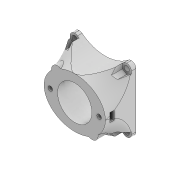
# Autodesk Inventor part: Female 22 to oxy
Saved by Autodesk Inventor 2020 (Build 240168000, 168)
## iProperties
Created: 2020-05-08
Part Number: Female 22 to oxy
Material: Generic
Document SubType Name: Modeling
Designer: rayan
Density: 1 g/cm^3
Appearance: Default
Author: rayan
Autodesk Inventor part; units mm, degrees
ref_plane "YZ Plane" through (0, 0, 0) normal (1, 0, 0) x (0, 1, 0)
ref_plane "XZ Plane" through (0, 0, 0) normal (0, 1, 0) x (-1, 0, 0)
ref_plane "XY Plane" through (0, 0, 0) normal (0, 0, 1) x (1, 0, 0)
sketch "Sketch3" plane through (0, 0, 0) normal (0, 0, 1) x (1, 0, 0)
  line L0 (-20.1, 21) -> (20.1, 21)
  line L1 (20.1, 21) -> (20.1, -21)
  line L2 (20.1, -21) -> (-20.1, -21)
  line L3 (-20.1, -21) -> (-20.1, 21)
  line L4 (-20.1, 21) -> (20.1, -21) construction
  line L5 (20.1, 21) -> (-20.1, -21) construction
  point P0 (0, 0)
  dimension "d24" = 40.2
  dimension "d25" = 42
  constraints: 12 end point, 2 midpoint, 2 parallel, 1 horizontal, 1 perpendicular
  measures "d24" distance of L1.end L2.end
  measures "d25" distance of L0.end L1.end
extrude "Extrusion3" add sketch "Sketch3" along normal blind 20
sketch "Sketch4" plane through (0, 0, 20) normal (0, 0, 1) x (1, 0, 0)
  line L0 (20.1, 21) -> (-20.1, 21) projected
  line L1 (-20.1, 21) -> (-17.1, 21) construction
  line L2 (-17.1, 21) -> (-17.1, 18) construction
  line L3 (-17.1, 18) -> (-20.1, 18) construction
  line L4 (-20.1, 18) -> (-20.1, 21) construction
  circle A0 centre (-17.1, 18) radius 1.7
  point P0 (0, 0)
  dimension "d28" = 3
  dimension "d29" = 3
  dimension "d30" = 3.4
  constraints: 8 end point, 2 parallel, 1 centre point, 1 coincident, 1 horizontal, 1 perpendicular
  measures "d28" distance of L2.end L3.end
  measures "d29" distance of L1.end L2.end
  measures "d30" diameter of A0
extrude "Extrusion4" cut sketch "Sketch4" against normal through all
fillet "Fillet2" radius 3 1 edges at (-20.1, 21, 10)
mirror "Mirror2" about plane through (0, 0, 0) normal (0, 1, 0) of "Fillet2", "Extrusion4"
mirror "Mirror3" about plane through (0, 0, 0) normal (1, 0, 0) of "Fillet2", "Extrusion4", "Mirror2"
sketch "Sketch5" plane through (0, 0, 20) normal (0, 0, 1) x (1, 0, 0)
  circle A0 centre (-17.1, 18) radius 1.7 construction
  circle A1 centre (17.1, 18) radius 1.7 construction
  line L0 (-17.1, 18) -> (17.1, 18) construction
  line L1 (17.1, 18) -> (17.1, 15) construction
  line L2 (17.1, 15) -> (-17.1, 15) construction
  line L3 (-17.1, 15) -> (-17.1, 18) construction
  arc A2 (-17.1, 21) -> (-20.1, 18) centre (-17.1, 18) ccw construction
  line L4 (-17.1, 18) -> (-17.1, 21) construction
  line L5 (17.1, 21) -> (-17.1, 21) construction
  line L6 (17.1, 18) -> (17.1, 21) construction
  line L7 (-17.1, 18) -> (-17.1, 21) construction
  line L8 (-17.1, 21) -> (-16, 21) construction
  line L9 (-16, 21) -> (-16, 18) construction
  line L10 (-16, 18) -> (-17.1, 18) construction
  line L11 (17.1, 18) -> (17.1, 21) construction
  line L12 (17.1, 21) -> (16, 21) construction
  line L13 (16, 21) -> (16, 18) construction
  line L14 (16, 18) -> (17.1, 18) construction
  arc A3 (-16, 21) -> (16, 21) centre (0, 39.3333) ccw
  line L15 (-16, 21) -> (16, 21)
  point P0 (0, 0)
  point P1 (0, 15)
  dimension "d34" = 3
  dimension "d87" = 1.1
  dimension "d88" = 1.1
  constraints: 30 end point, 7 equal length, 5 perpendicular, 3 point on circle, 2 vertical, 1 centre point, 1 horizontal, 1 midpoint
  measures "d34" distance of L0.end L1.end
  measures "d87" distance of L4.end L8.end
  measures "d88" distance of L13.end L0.end
extrude "Extrusion5" cut sketch "Sketch5" against normal through all
mirror "Mirror4" about plane through (0, 0, 0) normal (0, 1, 0) of "Extrusion5"
fillet "Fillet3" radius 3 4 edges at (16, 21, 10) (-16, 21, 10) (-16, -21, 10) (16, -21, 10)
sketch "Sketch7" plane through (0, 0, 20) normal (0, 0, 1) x (1, 0, 0)
  line L0 (15.3, 7.9) -> (15.3, -11.6) construction
  line L1 (15.3, -11.6) -> (-15.4, -11.6) construction
  line L2 (-15.4, -11.6) -> (-15.4, 7.9) construction
  line L3 (-15.4, 7.9) -> (15.3, 7.9) construction
  line L4 (-17.65, -15) -> (30.6, -15) construction
  line L5 (30.6, -15) -> (30.6, 15) construction
  line L6 (30.6, 15) -> (-30.1, 15) construction
  line L7 (-30.1, 15) -> (-30.1, 10) construction
  line L8 (-17.65, 10) -> (-30.1, 10) construction
  line L9 (-17.65, 10) -> (-17.65, -15) construction
  line L10 (15.3, -11.6) -> (-15.4, 7.9) construction
  line L11 (-15.4, -11.6) -> (15.3, 7.9) construction
  line L12 (0, 0) -> (-0.05, 0) construction
  line L13 (-0.05, 0) -> (-0.05, -1.85) construction
  line L14 (-0.05, -1.85) -> (0, -1.85) construction
  line L15 (0, -1.85) -> (0, 0) construction
  circle A0 centre (0, -1.85) radius 9
  dimension "d41" = 18
  constraints: 12 end point, 2 parallel, 1 centre point, 1 coincident, 1 horizontal, 1 midpoint, 1 perpendicular
  measures "d41" diameter of A0
extrude "Extrusion6" cut sketch "Sketch7" against normal through all
sketch "Sketch8" plane through (0, 0, 0) normal (1, 0, 0) x (0, 1, 0)
  line L0 (7.15, 0) -> (-10.85, 0) projected
  line L1 (-10.85, 20) -> (7.15, 20) projected
  line L2 (-18, 0) -> (18, 0) projected
  line L3 (-18, 20) -> (18, 20) projected
  line L4 (-1.45, 0) -> (-1.45, 20)
  line L5 (-1.45, 20) -> (9.55, 20)
  line L6 (9.55, 20) -> (9.55, 0) construction
  line L7 (9.55, 0) -> (-1.45, 0)
  line L8 (0, 0) -> (-1.45, 0)
  line L9 (9.55, 0) -> (9.55, 20) construction
  line L10 (9.55, 20) -> (9.8, 20) construction
  line L11 (9.8, 20) -> (9.8, 0) construction
  line L12 (9.8, 0) -> (9.55, 0) construction
  line L13 (9.55, 0) -> (9.8, 20)
  line L14 (9.55, 20) -> (9.8, 20)
  point P0 (-17.2722, 0)
  point P1 (17.2722, 0)
  point P2 (-17.2722, 20)
  point P3 (17.2722, 20)
  point P4 (9.8, 20)
  dimension "d42" = 11
  dimension "d43" = 0.25
  constraints: 22 end point, 4 parallel, 3 collinear, 3 perpendicular, 2 point on line
  measures "d42" distance of L4.end L5.end
  measures "d43" distance of L5.end L10.end
revolve "Revolution1" cut sketch "Sketch8" angle 360 about axis through (0, -1.45, 0) along (0, 0, 1)
sketch "Sketch9" plane through (0, 0, 20) normal (0, 0, 1) x (1, 0, 0)
  line L0 (6.3337, 11.8636) -> (-10.8812, 11.8636) construction
  line L1 (-10.8812, 11.8636) -> (-10.8812, 17.151) construction
  line L2 (-10.8812, 17.151) -> (6.3337, 17.151) construction
  line L3 (6.3337, 17.151) -> (6.3337, 11.8636) construction
  point P0 (0, 0)
  constraints: 2 other
extrude "Extrusion7" [suppressed]
ref_plane "Work Plane1" through (0, 0, 3) normal (0, 0, -1) x (-1, 0, 0)
sketch "Sketch10" plane through (0, 0, 3) normal (0, 0, -1) x (-1, 0, 0)
  circle A0 centre (-17.1, -18) radius 1.7 construction
  line L0 (-17.1, -18) -> (-17.1, -23.7125) construction
  line L1 (-17.1, -21.3486) -> (-20, -19.6743) construction
  line L2 (-20, -19.6743) -> (-20, -16.3257) construction
  line L3 (-20.1, -16.3834) -> (-17.1, -14.6514)
  line L4 (-17.1, -14.6514) -> (-14.2, -16.3257)
  line L5 (-14.2, -16.3257) -> (-14.2, -19.6743)
  line L6 (-14.2, -19.6743) -> (-17.1, -21.3486) construction
  line L7 (-14.2, -19.6743) -> (-20, -19.6743) construction
  line L8 (-20, -19.6743) -> (-20, -21.4064) construction
  line L9 (-20, -21.4064) -> (-14.2, -21.4064)
  line L10 (-14.2, -21.4064) -> (-14.2, -19.6743)
  circle A1 centre (0, -1.45) radius 11 construction
  arc A2 (-17.088, -21) -> (-15.2125, -20.3415) centre (-17.088, -18) ccw construction
  arc A3 (15.2125, -20.3415) -> (-15.2125, -20.3415) centre (0, -39.3333) ccw construction
  arc A4 (15.2125, -20.3415) -> (17.088, -21) centre (17.088, -18) ccw construction
  line L11 (17.1, -21) -> (17.088, -21) construction
  arc A5 (17.1, -21) -> (20.1, -18) centre (17.1, -18) ccw construction
  line L12 (20.1, 18) -> (20.1, -18) construction
  arc A6 (20.1, 18) -> (17.1, 21) centre (17.1, 18) ccw construction
  line L13 (17.088, 21) -> (17.1, 21) construction
  arc A7 (17.088, 21) -> (15.2125, 20.3415) centre (17.088, 18) ccw construction
  arc A8 (-15.2125, 20.3415) -> (15.2125, 20.3415) centre (0, 39.3333) ccw construction
  arc A9 (-15.2125, 20.3415) -> (-17.088, 21) centre (-17.088, 18) ccw construction
  line L14 (-17.1, 21) -> (-17.088, 21) construction
  arc A10 (-17.1, 21) -> (-20.1, 18) centre (-17.1, 18) ccw construction
  line L15 (-20.1, -18) -> (-20.1, 18) construction
  arc A11 (-20.1, -18) -> (-17.1, -21) centre (-17.1, -18) ccw construction
  line L16 (-17.088, -21) -> (-17.1, -21) construction
  circle A12 centre (-17.1, 18) radius 1.7 construction
  circle A13 centre (17.1, 18) radius 1.7 construction
  circle A14 centre (17.1, -18) radius 1.7 construction
  circle A15 centre (-17.1, -18) radius 1.7 construction
  line L17 (-20.1, -16.3834) -> (-20, -16.3834) construction
  line L18 (-20, -16.3834) -> (-20, -21.4064) construction
  line L19 (-20, -21.4064) -> (-20.1, -21.4064)
  line L20 (-20.1, -21.4064) -> (-20.1, -16.3834)
  point P0 (0, 0)
  dimension "d48" = 5.8
  constraints: 30 end point, 4 parallel, 3 point on line, 2 horizontal, 2 perpendicular, 1 coincident, 1 vertical, 13 other
  measures "d48" distance between parallel lines of L2 L5
extrude "Extrusion8" cut sketch "Sketch10" against normal through all
mirror "Mirror5" about plane through (0, 0, 0) normal (0, 1, 0) of "Extrusion8"
mirror "Mirror6" about plane through (0, 0, 0) normal (1, 0, 0) of "Extrusion8", "Mirror5"
sketch "Sketch11" plane through (0, 0, 20) normal (0, 0, 1) x (1, 0, 0)
  circle A0 centre (0, -1.45) radius 11.25 projected
  line L0 (0, -1.45) -> (16, -1.45)
  line L1 (20.1, -18) -> (20.1, 18) projected
  circle A1 centre (16, -1.45) radius 1.5
  point P0 (0, 0)
  point P1 (20.1, -17.2722)
  point P2 (20.1, 17.2722)
  dimension "d51" = 16
  dimension "d52" = 3
  constraints: 2 end point, 1 centre point, 1 coincident, 1 perpendicular
  measures "d51" distance of L0.start L0.end
  measures "d52" diameter of A1
extrude "Extrusion9" cut sketch "Sketch11" against normal blind 10 contours A1
ref_plane "Work Plane2" through (0, 0, 17) normal (0, 0, 1) x (1, 0, 0)
sketch "Sketch12" plane through (0, 0, 17) normal (0, 0, 1) x (1, 0, 0)
  circle A0 centre (16, -1.45) radius 1.5 projected
  line L0 (16, -1.45) -> (21, -1.45)
  line L1 (19.3486, -1.45) -> (17.6743, -4.35) construction
  line L2 (17.6743, -4.35) -> (14.3257, -4.35)
  line L3 (14.3257, -4.35) -> (12.6514, -1.45)
  line L4 (12.6514, -1.45) -> (14.3257, 1.45)
  line L5 (14.3257, 1.45) -> (17.6743, 1.45)
  line L6 (17.6743, 1.45) -> (19.3486, -1.45) construction
  line L7 (17.6743, -4.35) -> (17.6743, 1.45) construction
  line L8 (17.6743, 1.45) -> (27.6743, 1.45)
  line L9 (27.6743, 1.45) -> (27.6743, -4.35)
  line L10 (27.6743, -4.35) -> (17.6743, -4.35)
  point P0 (0, 0)
  point P1 (16, -1.85)
  dimension "d111" = 5
  dimension "d112" = 5.8
  dimension "d113" = 10
  constraints: 22 end point, 2 parallel, 2 perpendicular, 1 coincident, 1 horizontal, 1 point on line, 13 other
  measures "d111" distance of L0.start L0.end
  measures "d112" distance between parallel lines of L2 L5
  measures "d113" distance of L9.end L1.end
extrude "Extrusion10" cut sketch "Sketch12" against normal blind 2.8
mirror "Mirror7" about plane through (0, 0, 0) normal (1, 0, 0) of "Extrusion10", "Extrusion9"
sketch "Sketch13" plane through (0, 0, 20) normal (0, 0, 1) x (1, 0, 0)
  circle A0 centre (-17.1, 18) radius 1.7 projected
  point P0 (0, 0)
extrude "Extrusion11" [suppressed]
mirror "Mirror8" [suppressed]
mirror "Mirror9" [suppressed]
sketch "Sketch14" plane through (0, 0, 0) normal (0, 0, -1) x (-1, 0, 0)
  line L0 (5.3455, 10.4926) -> (-17.7314, 10.4926) construction
  line L1 (-17.7314, 10.4926) -> (-17.7314, 22.1476) construction
  line L2 (-17.7314, 22.1476) -> (5.3455, 22.1476) construction
  line L3 (5.3455, 22.1476) -> (5.3455, 10.4926) construction
  spline S0 degree 2 poles (2.9398, 12.6949) (2.9398, 12.8381) (3.0114, 13.0787) (3.1432, 13.2734) (3.3293, 13.4166) (3.5613, 13.5169) (3.8276, 13.5656) (3.9995, 13.5656) knots 0 0 0 1 2 3 4 5 6 6 6
  line L4 (3.9995, 13.5656) -> (4.7927, 13.5656)
  spline S1 degree 2 poles (4.7927, 13.5656) (4.8443, 13.5656) (4.9417, 13.494) (4.9417, 13.4023) knots 0 0 0 1 2 2 2
  line L5 (4.9417, 13.4023) -> (4.9417, 10.6931)
  spline S2 degree 2 poles (4.9417, 10.6931) (4.9417, 10.6015) (4.8443, 10.5299) (4.7927, 10.5299) knots 0 0 0 1 2 2 2
  line L6 (4.7927, 10.5299) -> (4.1025, 10.5299)
  spline S3 degree 2 poles (4.1025, 10.5299) (3.8276, 10.5299) (3.4811, 10.633) (3.2491, 10.8306) (3.1317, 11.117) (3.1317, 11.2974) knots 0 0 0 1 2 3 4 4 4
  spline S4 degree 2 poles (3.1317, 11.2974) (3.1317, 11.4062) (3.1833, 11.601) (3.2835, 11.7699) (3.4381, 11.8988) (3.5355, 11.9417) knots 0 0 0 1 2 3 4 4 4
  spline S5 degree 2 poles (3.5355, 11.9417) (3.4124, 11.9647) (3.1947, 12.0907) (3.0343, 12.2825) (2.9398, 12.5403) (2.9398, 12.6949) knots 0 0 0 1 2 3 4 4 4
  spline S6 degree 2 poles (3.3637, 12.7179) (3.3637, 12.5833) (3.4496, 12.3771) (3.6157, 12.2339) (3.8677, 12.1623) (4.0567, 12.1623) knots 0 0 0 1 2 3 4 4 4
  line L7 (4.0567, 12.1623) -> (4.5407, 12.1623)
  line L8 (4.5407, 12.1623) -> (4.5407, 13.2333)
  line L9 (4.5407, 13.2333) -> (3.9536, 13.2333)
  spline S7 degree 2 poles (3.9536, 13.2333) (3.8162, 13.2333) (3.61, 13.1675) (3.4525, 13.0386) (3.3637, 12.8467) (3.3637, 12.7179) knots 0 0 0 1 2 3 4 4 4
  spline S8 degree 2 poles (3.547, 11.3375) (3.547, 11.2286) (3.6071, 11.0482) (3.7388, 10.9251) (3.9508, 10.8592) (4.1226, 10.8592) knots 0 0 0 1 2 3 4 4 4
  line L10 (4.1226, 10.8592) -> (4.5407, 10.8592)
  line L11 (4.5407, 10.8592) -> (4.5407, 11.8415)
  line L12 (4.5407, 11.8415) -> (4.0825, 11.8415)
  spline S9 degree 2 poles (4.0825, 11.8415) (3.925, 11.8415) (3.7331, 11.7585) (3.6042, 11.621) (3.547, 11.4348) (3.547, 11.3375) knots 0 0 0 1 2 3 4 4 4
  spline S10 degree 2 poles (0.0531, 13.4224) (0.0359, 13.4739) (0.033, 13.5369) (0.0702, 13.5713) (0.1562, 13.5799) (0.2306, 13.5799) knots 0 0 0 1 2 3 4 4 4
  spline S11 degree 2 poles (0.2306, 13.5799) (0.3022, 13.5799) (0.3881, 13.5741) (0.434, 13.557) (0.454, 13.5283) (0.4655, 13.5083) knots 0 0 0 1 2 3 4 4 4
  line L13 (0.4655, 13.5083) -> (0.7232, 12.7694)
  line L14 (0.7232, 12.7694) -> (1.9862, 12.7694)
  line L15 (1.9862, 12.7694) -> (2.2353, 13.4968)
  spline S12 degree 2 poles (2.2353, 13.4968) (2.2439, 13.5197) (2.2668, 13.5484) (2.3098, 13.5713) (2.3928, 13.5799) (2.4587, 13.5799) knots 0 0 0 1 2 3 4 4 4
  spline S13 degree 2 poles (2.4587, 13.5799) (2.5274, 13.5799) (2.6133, 13.5684) (2.6477, 13.534) (2.6448, 13.471) (2.6277, 13.4195) knots 0 0 0 1 2 3 4 4 4
  line L16 (2.6277, 13.4195) -> (1.6081, 10.6015)
  spline S14 degree 2 poles (1.6081, 10.6015) (1.5995, 10.5728) (1.568, 10.5413) (1.5108, 10.5213) (1.4191, 10.5156) (1.3475, 10.5156) knots 0 0 0 1 2 3 4 4 4
  spline S15 degree 2 poles (1.3475, 10.5156) (1.2731, 10.5156) (1.1757, 10.5213) (1.1127, 10.5413) (1.0812, 10.5757) (1.0726, 10.6015) knots 0 0 0 1 2 3 4 4 4
  line L17 (1.0726, 10.6015) -> (0.0531, 13.4224)
  line L18 (1.359, 10.9337) -> (1.3618, 10.9337)
  line L19 (1.3618, 10.9337) -> (1.8859, 12.4486)
  line L20 (1.8859, 12.4486) -> (0.8292, 12.4486)
  line L21 (0.8292, 12.4486) -> (1.359, 10.9337)
  spline S16 degree 2 poles (-2.4814, 13.1331) (-2.4814, 13.1703) (-2.4757, 13.2276) (-2.4643, 13.2706) (-2.4471, 13.3021) (-2.3984, 13.3508) (-2.2495, 13.4453) (-2.0261, 13.5398) (-1.7368, 13.6028) (-1.565, 13.6028) knots 0 0 0 1 2 3 4 5 6 7 8 8 8
  spline S17 degree 2 poles (-1.565, 13.6028) (-1.27, 13.6028) (-0.7918, 13.4052) (-0.4567, 13.0214) (-0.2763, 12.4544) (-0.2763, 12.0878) knots 0 0 0 1 2 3 4 4 4
  spline S18 degree 2 poles (-0.2763, 12.0878) (-0.2763, 11.7098) (-0.471, 11.1198) (-0.8233, 10.7074) (-1.3159, 10.4926) (-1.6137, 10.4926) knots 0 0 0 1 2 3 4 4 4
  spline S19 degree 2 poles (-1.6137, 10.4926) (-1.7454, 10.4926) (-1.9946, 10.5413) (-2.2036, 10.6158) (-2.3698, 10.716) (-2.4328, 10.779) (-2.4499, 10.8105) (-2.4643, 10.8563) (-2.47, 10.9165) (-2.47, 10.9594) knots 0 0 0 1 2 3 4 5 6 7 8 8 8
  spline S20 degree 2 poles (-2.47, 10.9594) (-2.47, 11.0053) (-2.4614, 11.0711) (-2.4413, 11.117) (-2.4156, 11.137) (-2.3955, 11.137) knots 0 0 0 1 2 3 4 4 4
  spline S21 degree 2 poles (-2.3955, 11.137) (-2.364, 11.137) (-2.2466, 11.0454) (-2.0576, 10.9365) (-1.7913, 10.8449) (-1.6051, 10.8449) knots 0 0 0 1 2 3 4 4 4
  spline S22 degree 2 poles (-1.6051, 10.8449) (-1.4018, 10.8449) (-1.0696, 11.0053) (-0.8319, 11.3203) (-0.703, 11.7728) (-0.703, 12.0649) knots 0 0 0 1 2 3 4 4 4
  spline S23 degree 2 poles (-0.703, 12.0649) (-0.703, 12.3513) (-0.829, 12.7952) (-1.061, 13.093) (-1.4018, 13.2448) (-1.6166, 13.2448) knots 0 0 0 1 2 3 4 4 4
  spline S24 degree 2 poles (-1.6166, 13.2448) (-1.7998, 13.2448) (-2.0719, 13.156) (-2.2609, 13.0443) (-2.3841, 12.9556) (-2.4213, 12.9556) knots 0 0 0 1 2 3 4 4 4
  spline S25 degree 2 poles (-2.4213, 12.9556) (-2.4356, 12.9556) (-2.4614, 12.9699) (-2.4757, 13.01) (-2.4814, 13.0787) (-2.4814, 13.1331) knots 0 0 0 1 2 3 4 4 4
  spline S26 degree 2 poles (-4.9988, 13.4997) (-4.9988, 13.5197) (-4.9816, 13.5484) (-4.9329, 13.5684) (-4.8556, 13.5799) (-4.7897, 13.5799) knots 0 0 0 1 2 3 4 4 4
  spline S27 degree 2 poles (-4.7897, 13.5799) (-4.7095, 13.5799) (-4.6064, 13.5656) (-4.5549, 13.5283) (-4.5377, 13.5054) knots 0 0 0 1 2 3 3 3
  line L22 (-4.5377, 13.5054) -> (-3.4208, 11.9876)
  line L23 (-3.4208, 11.9876) -> (-3.4208, 13.5054)
  spline S28 degree 2 poles (-3.4208, 13.5054) (-3.4208, 13.5226) (-3.4007, 13.5512) (-3.3549, 13.5684) (-3.2776, 13.5799) (-3.2203, 13.5799) knots 0 0 0 1 2 3 4 4 4
  spline S29 degree 2 poles (-3.2203, 13.5799) (-3.163, 13.5799) (-3.0829, 13.5684) (-3.037, 13.5512) (-3.017, 13.5226) (-3.017, 13.5054) knots 0 0 0 1 2 3 4 4 4
  line L24 (-3.017, 13.5054) -> (-3.017, 10.59)
  spline S30 degree 2 poles (-3.017, 10.59) (-3.017, 10.5728) (-3.037, 10.5442) (-3.0829, 10.527) (-3.163, 10.5156) (-3.2203, 10.5156) knots 0 0 0 1 2 3 4 4 4
  spline S31 degree 2 poles (-3.2203, 10.5156) (-3.2776, 10.5156) (-3.3549, 10.527) (-3.4007, 10.5442) (-3.4208, 10.5728) (-3.4208, 10.59) knots 0 0 0 1 2 3 4 4 4
  line L25 (-3.4208, 10.59) -> (-3.4208, 11.9389)
  line L26 (-3.4208, 11.9389) -> (-4.4947, 10.59)
  spline S32 degree 2 poles (-4.4947, 10.59) (-4.509, 10.57) (-4.5463, 10.5413) (-4.6007, 10.5241) (-4.678, 10.5156) (-4.7382, 10.5156) knots 0 0 0 1 2 3 4 4 4
  spline S33 degree 2 poles (-4.7382, 10.5156) (-4.8012, 10.5156) (-4.8756, 10.527) (-4.9214, 10.5471) (-4.9358, 10.5728) (-4.9358, 10.59) knots 0 0 0 1 2 3 4 4 4
  spline S34 degree 2 poles (-4.9358, 10.59) (-4.9358, 10.6215) (-4.9071, 10.6817) (-4.8642, 10.7361) knots 0 0 0 1 2 2 2
  line L27 (-4.8642, 10.7361) -> (-3.8561, 11.9389)
  line L28 (-3.8561, 11.9389) -> (-4.9415, 13.3794)
  spline S35 degree 2 poles (-4.9415, 13.3794) (-4.9816, 13.4424) (-4.9988, 13.4854) (-4.9988, 13.4997) knots 0 0 0 1 2 2 2
  point P0 (0, 0)
  constraints: 2 other
extrude "Extrusion12" cut sketch "Sketch14" against normal blind 0.5
sketch "Sketch26" plane through (0, 0, 20) normal (0, 0, 1) x (1, 0, 0)
  circle A0 centre (-16, -1.45) radius 1.5 projected
  circle A1 centre (16, -1.45) radius 1.5 projected
  line L0 (-20.1, 16.3834) -> (-20.1, -16.3834) projected
  arc A2 (14.2, -19.573) -> (-14.2, -19.573) centre (0, -39.3333) ccw projected
  line L1 (20.1, -16.3834) -> (20.1, 16.3834) projected
  arc A3 (-14.2, 19.573) -> (14.2, 19.573) centre (0, 39.3333) ccw projected
  circle A4 centre (0, -1.45) radius 11.25 construction
  line L2 (-16, -1.45) -> (-20.1, -1.45)
  ellipse E0 centre (0, -1.45) end of major axis (-20.1, -1.45) minor radius 16.45
  line L3 (-20.1, 16.3834) -> (-20.1, -16.3834) projected
  arc A5 (-14.2, 19.573) -> (14.2, 19.573) centre (0, 39.3333) ccw projected
  arc A6 (14.2, -19.573) -> (-14.2, -19.573) centre (0, -39.3333) ccw projected
  line L4 (0, -15) -> (0, -17.9) construction
  line L5 (-17.1, 14.6514) -> (-20.1, 16.3834) projected
  line L6 (-20.1, -16.3834) -> (-17.1, -14.6514) projected
  line L7 (-17.1, -14.6514) -> (-14.2, -16.3257) projected
  line L8 (-14.2, -16.3257) -> (-14.2, -19.573) projected
  line L9 (14.2, -19.573) -> (14.2, -16.3257) projected
  line L10 (14.2, -16.3257) -> (17.1, -14.6514) projected
  line L11 (17.1, -14.6514) -> (20.1, -16.3834) projected
  line L12 (20.1, 16.3834) -> (17.1, 14.6514) projected
  line L13 (17.1, 14.6514) -> (14.2, 16.3257) projected
  line L14 (14.2, 16.3257) -> (14.2, 19.573) projected
  line L15 (-14.2, 19.573) -> (-14.2, 16.3257) projected
  line L16 (-14.2, 16.3257) -> (-17.1, 14.6514) projected
  point P0 (0, 0)
  point P1 (0, 15)
  point P2 (0, 15)
  point P3 (20.1, -1.45)
  point P4 (-8.2627, -16.4458)
  point P5 (8.2627, -16.4458)
  constraints: 4 end point, 4 point on circle, 2 vertical, 1 coincident, 1 perpendicular, 1 point on line, 5 other
sketch "Sketch27" plane through (20.1, -18, 0) normal (1, 0, 0) x (0, 0, -1)
  line L0 (-20, 15.05) -> (-20, 18.05) projected
  line L1 (-20, 39) -> (0, 39) projected
  arc A0 (-20, 16.55) -> (-3, 39) centre (-27.9689, 40.2459) ccw
  point P0 (0, 18)
  dimension "d92" = 25
  constraints: 2 point on circle, 1 centre point, 1 midpoint
  measures "d92" radius of A0
sweep "Sweep4" cut profiles "Sketch26" path "Sketch27" keep normal constant yes path curves A0 contours L5 L16 L15 A3 E0 L0 | A3 L14 L13 L12 L1 E0
sketch "Sketch29" plane through (0, 0, 0) normal (1, 0, 0) x (0, 1, 0)
  line L0 (-15, 0) -> (-15, 20) construction
  line L1 (15, 20) -> (-17.9, 20) construction
  line L2 (-15, 20) -> (-17.9, 20) construction
  line L3 (-15, 0) -> (-20.3415, 0) construction
  line L4 (-15, 0) -> (-17.9, 20)
  point P0 (0, 0)
  constraints: 2 end point
sweep "Sweep5" add profiles "Sketch26" path "Sketch29" keep normal constant yes picked at (0.9346, -16.8782) contours A2 E0
sketch "Sketch30" plane through (-20.1, -18, 0) normal (-1, 0, 0) x (0, 0, 1)
  line L0 (20, 16.55) -> (20, 1.6166) construction
  line L1 (3, 0) -> (3, -3) projected
  arc A0 (20, 16.55) -> (3, -3) centre (22.9987, -3.2239) ccw
  point P0 (0, 18)
  dimension "d98" = 20
  constraints: 2 point on circle, 1 centre point
  measures "d98" radius of A0
sketch "Sketch31" plane through (0, 0, 20) normal (0, 0, 1) x (1, 0, 0)
  ellipse E0 centre (0, -1.45) end of major axis (20.1, -1.45) minor radius 16.45 (0, 15) -> (-20.1, -1.45) ccw projected
  line L0 (-20.1, -1.45) -> (-20.1, -16.3834) projected
  line L1 (-20.1, -16.3834) -> (-17.1, -14.6514) projected
  line L2 (-17.1, -14.6514) -> (-14.2, -16.3257) projected
  line L3 (-14.2, -16.3257) -> (-14.2, -19.573) projected
  arc A0 (-8.2627, -16.4458) -> (-14.2, -19.573) centre (0, -39.3333) ccw projected
  ellipse E1 centre (0, -1.45) end of major axis (-20.1, -1.45) minor radius 16.45 (-8.2627, -16.4458) -> (8.2627, -16.4458) ccw projected
  arc A1 (14.2, -19.573) -> (8.2627, -16.4458) centre (0, -39.3333) ccw projected
  line L4 (14.2, -19.573) -> (14.2, -16.3257) projected
  line L5 (14.2, -16.3257) -> (17.1, -14.6514) projected
  line L6 (17.1, -14.6514) -> (20.1, -16.3834) projected
  line L7 (20.1, -16.3834) -> (20.1, -1.45) projected
  ellipse E2 centre (0, -1.45) end of major axis (20.1, -1.45) minor radius 16.45 (20.1, -1.45) -> (0, 15) ccw projected
  circle A2 centre (-16, -1.45) radius 1.5 projected
  circle A3 centre (16, -1.45) radius 1.5 projected
  circle A4 centre (0, -1.45) radius 11.25 projected
  ellipse E3 centre (0, -1.45) end of major axis (20.1, -1.45) minor radius 16.45 (0, 15) -> (-20.1, -1.45) ccw projected
  ellipse E4 centre (0, -1.45) end of major axis (20.1, -1.45) minor radius 16.45
  point P0 (0, 0)
  point P1 (8.2627, -16.4458)
  point P2 (-8.2627, -16.4458)
  constraints: 1 coincident, 8 other
sketch "Sketch32" plane through (-20.1, -18, 0) normal (-1, 0, 0) x (0, 0, 1)
  line L0 (3, -1.7) -> (3, 1.7) construction
  line L1 (3, 0) -> (3, 0) construction
  line L2 (3, -2.3415) -> (3, -3) construction
  line L3 (3, -1.573) -> (3, -2.3415) construction
  line L4 (3, -1.573) -> (3, 1.6743) construction
  line L5 (3, 1.6743) -> (3, 3.3486) construction
  line L6 (3, 3.3486) -> (3, 1.6166) construction
  line L7 (3, 0) -> (3, 1.6166) construction
  line L8 (20, 33) -> (20, 16.55) construction
  line L9 (20, 16.55) -> (20, 1.6166) construction
  line L10 (20, 1.6166) -> (20, 3.3486) construction
  line L11 (20, 3.3486) -> (20, 1.6743) construction
  line L12 (20, 1.6743) -> (20, -1.573) construction
  line L13 (20, -1.573) -> (20, 1.5542) construction
  line L14 (20, 1.5542) -> (20, 1.5542) construction
  line L15 (20, 1.5542) -> (20, -1.573) construction
  line L16 (20, -1.573) -> (20, 1.6743) construction
  line L17 (20, 1.6743) -> (20, 3.3486) construction
  line L18 (20, 3.3486) -> (20, 1.6166) construction
  line L19 (20, 1.6166) -> (20, 16.55) construction
  line L20 (20, 16.55) -> (20, 33) construction
  line L21 (20, 18.05) -> (20, 15.05) construction
  line L22 (20, 18.05) -> (20, 15.05) construction
  line L23 (20, 27.8) -> (20, 5.3) construction
  line L24 (3, 0) -> (3, 0) projected
  arc A0 (20, 16.55) -> (3, 0) centre (22.7321, -3.2625) ccw
  point P0 (0, 18)
  dimension "d99" = 20
  constraints: 2 point on circle, 1 centre point
  measures "d99" radius of A0
sweep "Sweep6" cut profiles "Sketch31" path "Sketch32" keep normal constant yes path curves A0 contours E4 A0 L3 L2 L1 L0 | L7 L6 L5 L4 A1 E4
revolve "Revolution2" cut sketch "Sketch8" angle 360 about axis through (0, -1.45, 0) along (0, 0, 1)
sketch "Sketch33" plane through (0, 0, 20) normal (0, 0, 1) x (1, 0, 0)
  arc A0 (-11.8464, 6.9114) -> (-14.5, -1.45) centre (0, -1.45) ccw projected
  arc A1 (-17.5, -1.45) -> (-14.5, -1.45) centre (-16, -1.45) ccw projected
  arc A2 (-14.1407, 8.8597) -> (-17.5, -1.45) centre (0, -1.45) ccw projected
  arc A3 (-11.8464, 6.9114) -> (-14.1407, 8.8597) centre (-11.3137, 9.8637) ccw projected
  arc A4 (14.1407, -11.7597) -> (17.5, -1.45) centre (0, -1.45) ccw projected
  arc A5 (11.8464, -9.8114) -> (14.1407, -11.7597) centre (11.3137, -12.7637) ccw projected
  arc A6 (11.8464, -9.8114) -> (14.5, -1.45) centre (0, -1.45) ccw projected
  arc A7 (17.5, -1.45) -> (14.5, -1.45) centre (16, -1.45) ccw projected
  line L0 (-25, 23.55) -> (-25, -26.45) projected
  line L1 (-25, -26.45) -> (25, -26.45) projected
  line L2 (25, -26.45) -> (25, 23.55) projected
  line L3 (25, 23.55) -> (-25, 23.55) projected
  circle A8 centre (0, -1.45) radius 11.25 projected
  circle A9 centre (11.3137, -12.7637) radius 4
  circle A10 centre (-11.3137, 9.8637) radius 4
  point P0 (0, 0)
  dimension "d103" = 8
  dimension "d104" = 8
  constraints: 2 centre point, 2 coincident
  measures "d103" diameter of A9
  measures "d104" diameter of A10
extrude "Extrusion14" add sketch "Sketch33" against normal blind 10 contours A3 A2 A10 A0 | A0 A10 A2 A3 | A5 A6 A9 A4 | A4 A9 A6 A5
equation "\"d88\" = d87"
equation "\"d104\" = d103"
body "Solid2"
